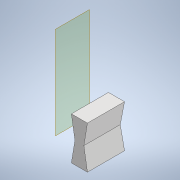
# Autodesk Inventor part: key
Saved by Autodesk Inventor 2022 (Build 260153000, 153)
## iProperties
Created: 2021-09-22
Part Number: key
Material: Generic
Document SubType Name: Modeling
Designer: tecware
Density: 1 g/cm^3
Appearance: Default
Author: tecware
## iProperties of the stored document key_3DPrint.ipt
Created: 2021-09-22
Part Number: key_3DPrint
Material: Generic
Document SubType Name: Modeling
Designer: tecware
Density: 1 g/cm^3
Appearance: Default
Author: tecware
Autodesk Inventor part; units mm, degrees
ref_plane "YZ Plane" through (0, 0, 0) normal (1, 0, 0) x (0, 1, 0)
ref_plane "XZ Plane" through (0, 0, 0) normal (0, 1, 0) x (-1, 0, 0)
sketch "Sketch1" plane through (0, 0, 0) normal (0, 0, 1) x (1, 0, 0)
  line L0 (10, -8) -> (-10, -8) projected
  line L1 (-7, -8) -> (-7.6667, -12)
  line L2 (-7.6667, -12) -> (-4.3333, -12)
  line L3 (-4.3333, -12) -> (-5, -8)
  line L4 (-6, -8) -> (-6.0726, -4.2007)
  line L5 (-6, -8) -> (-6.8, -8)
  line L6 (-6, -8) -> (-5.2, -8)
  line L7 (-6.8, -8) -> (-7.4332, -4.2007)
  line L8 (-7.4332, -4.2007) -> (-6.0726, -4.2007)
  line L9 (-5.2, -8) -> (-4.5668, -4.2007)
  line L10 (-4.5668, -4.2007) -> (-6.0726, -4.2007)
  line L11 (-6, -8) -> (-6.0726, -11.7993)
  line L12 (-6.8, -8) -> (-7.4332, -11.7993)
  line L13 (-7.4332, -11.7993) -> (-6.0726, -11.7993)
  line L14 (-5.2, -8) -> (-4.5668, -11.7993)
  line L15 (-4.5668, -11.7993) -> (-6.0726, -11.7993)
  line L16 (-7, -8) -> (-7.6667, -4)
  line L17 (-7.6667, -4) -> (-4.3333, -4)
  line L18 (-4.3333, -4) -> (-5, -8)
  point P0 (0, 0)
  point P1 (-8, -8)
  point P2 (-5.2, -8)
  dimension "d2" = 3.8
  dimension "d3" = 0.8
  dimension "d4" = 0.8
  constraints: 36 end point, 2 horizontal, 2 symmetric about line
  measures "d2" distance of L4.start L4.end
  measures "d3" distance of L4.start L5.end
  measures "d4" distance of L4.start L6.end
ref_plane "Work Plane1" through (-10, -8, -5.5) normal (0, 0, -1) x (0, 1, 0)
extrude "Extrusion1" add sketch "Sketch1" against normal blind 7 contours L14 L15 L11 L0 | L0 L4 L10 L9 | L11 L13 L12 L0 | L0 L7 L8 L4
ref_plane "Work Plane2" through (-10, -8, 0) normal (-1, 0, 0) x (0, 1, 0)
sketch "Sketch2" plane through (-10, -8, 0) normal (-1, 0, 0) x (0, 1, 0)
  line L0 (3.7993, 0) -> (3.7993, 7) projected
  line L1 (0, 0) -> (0, 7) projected
  line L2 (-3.7993, 0) -> (-3.7993, 7) projected
  line L3 (15, 7) -> (0, 6.5) projected
  line L4 (0, 7) -> (3.7993, 7) projected
  line L5 (3.7993, 7) -> (0, 7)
  line L6 (-3.7993, 0) -> (-3.7993, 7)
  line L7 (-15, 7) -> (0, 6.5)
  line L8 (0, 7) -> (-3.7993, 7)
  point P0 (8, 0)
  point P1 (-3.7993, 6.6266)
  point P2 (3.7993, 6.6266)
  constraints: 8 end point, 1 collinear, 1 symmetric about line
extrude "Extrusion2" cut sketch "Sketch2" against normal through all
body "Solid1"
